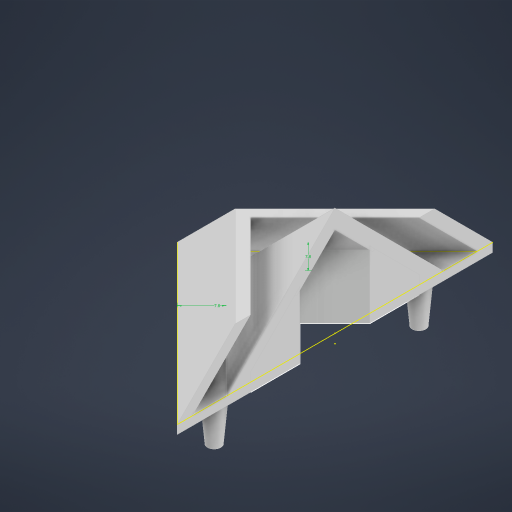
# Autodesk Inventor part: coltar5mmV3_notop
Saved by Autodesk Inventor 2023 (Build 270158000, 158)
## iProperties
Created: 2022-02-13
Part Number: coltar5mmV3_notop
Material: Generic
Document SubType Name: Modeling
Designer: Vlasciar
Density: 1 g/cm^3
Appearance: Default
Author: Vlasciar
Autodesk Inventor part; units mm, degrees
ref_plane "YZ Plane" through (0, 0, 0) normal (1, 0, 0) x (0, 1, 0)
ref_plane "XZ Plane" through (0, 0, 0) normal (0, 1, 0) x (-1, 0, 0)
ref_plane "XY Plane" through (0, 0, 0) normal (0, 0, 1) x (1, 0, 0)
sketch "Sketch2" plane through (0, 0, 0) normal (0, 1, 0) x (-1, 0, 0)
  line L0 (0, 35.355) -> (35.3557, 0)
  line L1 (35.3557, 0) -> (0, -35.355)
  line L2 (0, -35.355) -> (0, 35.355)
  point P0 (0, 0)
  point P1 (0, 0)
  dimension "d1" = 50
  dimension "d41" = 70.71
  constraints: 6 end point, 1 coincident, 1 equal length, 1 horizontal alignment, 1 midpoint
  measures "d1" distance of L0.start L0.end
  measures "d41" distance of L1.end L0.start
extrude "Extrusion1" add sketch "Sketch2" against normal blind 2
sketch "Sketch3" plane through (0, 0, 0) normal (0, 1, 0) x (1, 0, 0)
  line L0 (-35.3557, 0) -> (0, -35.355) projected
  line L1 (0, -35.355) -> (0, 35.355) projected
  line L2 (0, 35.355) -> (-35.3557, 0) projected
  point P0 (0, 0)
sketch "Sketch12" plane through (0, 0, 35.355) normal (1, 0, 0) x (0, 0, -1)
  line L0 (0, 0) -> (70.71, 0) projected
  line L1 (0, 0) -> (35.355, 35.3557)
  line L2 (35.355, 35.3557) -> (70.71, 0)
  line L3 (11.0308, 0) -> (59.6792, 0)
  line L4 (59.6792, 0) -> (35.355, 24.3247)
  line L5 (35.355, 24.3247) -> (11.0308, 0)
  point P0 (35.355, 0)
  point P1 (11.0308, 0)
  point P2 (59.6792, 0)
  dimension "d42" = 50
  dimension "d43" = 50
  dimension "d46" = 0
  dimension "d47" = 7.8
  dimension "d48" = 7.8
  constraints: 10 end point, 2 parallel, 1 horizontal
  measures "d42" distance of L1.end L0.end
  measures "d43" distance of L0.start L1.end
  measures "d46" distance between parallel lines of L0 L3
  measures "d47" distance between parallel lines of L2 L4
  measures "d48" distance between parallel lines of L1 L5
ref_plane "Work Plane5" through (-35.3557, 0, 0) normal (-0.5773466, 0.5773466, 0.5773577) x (0.7071136, 0, 0.7071)
ref_plane "Work Plane6" through (0, 0, -35.355) normal (0.5773466, -0.5773466, 0.5773577) x (-0.7071136, 0, 0.7071)
extrude "Extrusion10" add sketch "Sketch12" along normal up to surface surface through (-35.3557, 0, 0) normal (-0.5773466, 0.5773466, 0.5773577)
split "Split3" plane through (0, 0, -35.355) removes the side toward (-0.5773466, 0.5773466, -0.5773577)
shell "Shell3" thickness 2 removed faces 1 at (0, 11.7852, 0)
sketch "Sketch13" plane through (0, 0, 31.8909) normal (0, 1, 0) x (1, 0, 0)
  line L0 (-31.8916, 31.8909) -> (0, 0) projected
  line L1 (0, 63.7819) -> (0, 0) projected
  line L2 (0, 63.7819) -> (-31.8916, 31.8909) projected
  line L3 (0, 67.2459) -> (0, -3.4641) projected
  line L4 (0, 7.5667) -> (-24.3247, 31.8909)
  line L5 (-24.3247, 31.8909) -> (0, 56.2152)
  line L6 (0, -3.4641) -> (-35.3557, 31.8909) projected
  line L7 (-35.3557, 31.8909) -> (0, 67.2459) projected
  point P0 (0, 31.8909)
  dimension "d52" = 7.8
  dimension "d53" = 7.8
  constraints: 4 end point, 2 parallel, 2 point on line
  measures "d52" distance between parallel lines of L4 L6
  measures "d53" distance between parallel lines of L7 L5
ref_plane "Work Plane9" through (0, 24.3247, 0) normal (0.5773466, -0.5773466, -0.5773577) x (0, -0.7071136, 0.7071)
ref_plane "Work Plane10" through (0, 0, -24.3242) normal (-0.5773466, 0.5773466, -0.5773577) x (0, 0.7071136, 0.7071)
extrude "Extrusion18" add sketch "Sketch12" against normal up to surface separate body contours L5 L4 L0 surface through (0, 0, -24.3242) normal (-0.5773466, 0.5773466, -0.5773577)
split "Split5" plane through (0, 24.3247, 0) removes the side toward (-0.5773466, 0.5773466, 0.5773577) bodies 2
shell "Shell5" thickness 2 removed faces 1 at (0, 8.1082, 0) bodies 2
sketch "Sketch25" plane through (0, -2, 0) normal (0, -1, 0) x (1, 0, 0)
  line L0 (-18.8606, 0) -> (0, 18.8602) projected
  line L1 (0, -35.355) -> (0, 35.355) projected
  line L2 (0, 35.355) -> (-35.3557, 0) projected
  line L3 (-35.3557, 0) -> (0, -35.355) projected
  line L4 (0, -35.355) -> (0, 35.355) projected
  line L5 (0, -18.8602) -> (-18.8606, 0) projected
  point P0 (0, 0)
extrude "Extrusion24" cut sketch "Sketch25" against normal blind 2 contours L5 L1 L3 L2 L0 bodies 1
sketch "Sketch27" plane through (0, 0, 0) normal (0, -1, 0) x (1, 0, 0)
  line L0 (0, 35.355) -> (0, 31.8909) projected
  line L1 (-35.3557, 0) -> (0, 35.355) projected
  line L2 (0, -35.355) -> (-35.3557, 0) projected
  line L3 (0, -31.8909) -> (0, -35.355) projected
  line L4 (0, 35.355) -> (0, -35.355)
  line L5 (0, 0) -> (-35.3557, 0) projected
  line L6 (-35.3557, 0) -> (0, -35.355)
  line L7 (-35.3557, 0) -> (0, 35.355)
  line L8 (0, 18.8602) -> (-18.8606, 0) projected
  line L9 (0, 18.8602) -> (-18.8606, 0)
  line L10 (0, 24.3242) -> (0, -24.3242) projected
  line L11 (-18.8606, 0) -> (0, -18.8602)
  line L12 (0, -18.8602) -> (0, -35.355)
  point P0 (0, 31.8909)
  constraints: 12 end point, 3 collinear
extrude "Extrusion25" add sketch "Sketch27" along normal blind 2 contours L0 L4 L8 L5 L1 | L5 L11 L4 L3 L2 bodies 1
sketch "Sketch28" plane through (0, 2, 18.8602) normal (0, 1, 0) x (1, 0, 0)
  line L0 (0, 0) -> (-18.8606, 18.8602) projected
  line L1 (0, 37.7204) -> (0, 0) projected
  line L2 (-18.8606, 18.8602) -> (0, 37.7204) projected
  point P0 (0, 18.8602)
extrude "Extrusion26" cut sketch "Sketch28" against normal blind 10 bodies 2 1
sketch "Sketch29" plane through (0, -2, 0) normal (0, -1, 0) x (1, 0, 0)
  circle A0 centre (-4.0983, 22.9586) radius 1.5
  circle A1 centre (-4.0983, -22.9586) radius 1.5
  line L0 (0, 0) -> (-31.8916, 0) projected
  circle A2 centre (-26.4317, 0) radius 1.5
  dimension "d116" = 3
  dimension "d117" = 3
  dimension "d118" = 3
  constraints: 3 centre point, 1 point on line
  measures "d116" diameter of A0
  measures "d117" diameter of A1
  measures "d118" diameter of A2
extrude "Extrusion27" add sketch "Sketch29" along normal blind 10 bodies 1
draft "FaceDraft3" angle 5 pull direction (0, -1, 0) faces at (-2.6177, -8.6667, 22.718) (-2.6177, -8.6667, -23.1992) (-24.9511, -8.6667, -0.2406) fixed edges at (-5.5983, -12, 22.9586) (-5.5983, -12, -22.9586) (-27.9317, -12, 0)
ref_plane "Work Plane12" through (-9.1346, 13, 9.7258) normal (0, -1, 0) x (0.7071136, 0, 0.7071)
ref_plane "Work Plane11" through (-9.1346, -2, 9.7258) normal (0, -1, 0) x (0.7071136, 0, 0.7071)
sketch "Sketch30" plane through (-9.1346, 13, 9.7258) normal (0, -1, 0) x (0.7071136, 0, 0.7071)
  line L0 (27.2074, 21.2846) -> (-35.8048, 21.2846)
  line L1 (-35.8048, 21.2846) -> (-35.8048, -39.2765)
  line L2 (-35.8048, -39.2765) -> (27.2074, -39.2765)
  line L3 (27.2074, -39.2765) -> (27.2074, 21.2846)
  point P0 (-0.4179, -13.3363)
  constraints: 8 end point, 2 parallel, 1 horizontal, 1 perpendicular
extrude "Extrusion28" cut sketch "Sketch30" against normal blind 30 bodies 1 2
sketch "Sketch31" plane through (0, -2, 0) normal (0, -1, 0) x (1, 0, 0)
  line L0 (0, -18.8602) -> (-18.8606, 0) projected
  line L1 (-18.8606, 0) -> (0, 18.8602) projected
  line L2 (0, 18.8602) -> (0, 7.8604) projected
  line L3 (0, 18.8602) -> (0, 7.8604)
  line L4 (-7.8606, 0) -> (0, 7.8604) projected
  line L5 (0, 7.8604) -> (-7.8606, 0)
  line L6 (0, -7.8604) -> (-7.8606, 0) projected
  line L7 (-7.8606, 0) -> (0, -7.8604)
  line L8 (0, -7.8604) -> (0, -18.8602)
  line L9 (-18.8606, 0) -> (0, -18.8602)
  line L10 (-18.8606, 0) -> (0, 18.8602)
  line L11 (-18.8606, 0) -> (-7.8606, 0)
  point P0 (0, 0)
  constraints: 14 end point, 2 point on line, 1 collinear, 1 horizontal, 1 parallel
extrude "Extrusion29" add sketch "Sketch31" against normal up to surface contours L1 L2 L4 L11 surface through (-6.9534, 6.9534, 6.9536) normal (0.5773466, -0.5773466, -0.5773577) bodies 1
extrude "Extrusion30" add sketch "Sketch31" against normal up to surface contours L0 L11 L6 L8 surface through (-11.0077, 11.0077, 1.1547) normal (-0.5773466, 0.5773466, -0.5773577) bodies 1
sketch "Sketch33" plane through (-24.3247, 0, 0) normal (-0.5773466, 0.5773466, 0.5773577) x (0.7071136, 0, 0.7071)
  line L0 (25.2079, 15.9216) -> (9.1925, 15.9216) projected
  line L1 (9.1925, 15.9216) -> (14.1925, 24.5819)
  line L2 (25.2079, 15.9216) -> (20.208, 24.5819)
  line L3 (20.208, 24.5819) -> (14.1925, 24.5819)
  point P0 (17.2003, 9.9304)
  dimension "d129" = 10
  constraints: 6 end point, 1 horizontal
  measures "d129" distance of L0.end L1.end
sketch "Sketch34" plane through (0, 0, -24.3242) normal (-0.5773466, 0.5773466, -0.5773577) x (-0.7071136, 0, 0.7071)
  line L0 (25.2075, 15.9216) -> (9.1921, 15.9216) projected
  line L1 (9.1921, 15.9216) -> (11.6416, 17.3358) projected
  line L2 (9.1921, 15.9216) -> (14.192, 24.5819)
  line L3 (14.192, 24.5819) -> (20.2074, 24.5819)
  line L4 (20.2074, 24.5819) -> (25.2075, 15.9216)
  line L5 (25.2072, 25.1681) -> (25.2075, 15.9216) projected
  line L6 (25.2075, 15.9216) -> (9.1921, 15.9216)
  point P0 (17.1997, 9.9304)
  dimension "d130" = 10
  constraints: 8 end point, 1 collinear, 1 horizontal, 1 perpendicular
  measures "d130" distance of L0.end L2.end
extrude "Extrusion31" add sketch "Sketch33" against normal blind 2.45 bodies 2
extrude "Extrusion32" add sketch "Sketch34" against normal blind 2.45 bodies 2
sketch "Sketch35" plane through (0, 0, 35.355) normal (1, 0, 0) x (0, 0, -1)
  line L0 (19.9835, 25.4931) -> (55.8628, 25.4931)
  line L1 (55.8628, 25.4931) -> (55.8628, -4.2384)
  line L2 (55.8628, -4.2384) -> (19.9835, -4.2384)
  line L3 (19.9835, -4.2384) -> (19.9835, 25.4931)
  point P0 (35.355, 0)
  constraints: 8 end point, 2 parallel, 1 horizontal, 1 perpendicular
extrude "Extrusion33" cut sketch "Sketch35" along normal blind 2.45 bodies 2
sketch "Sketch37" plane through (0, 0, -24.3242) normal (-0.5773466, 0.5773466, -0.5773577) x (-0.7071136, 0, 0.7071)
  line L0 (20.2074, 24.5819) -> (14.192, 24.5819) projected
  line L1 (14.192, 24.5819) -> (17.8949, 30.9957)
  line L2 (20.2074, 24.5819) -> (16.715, 30.631)
  point P0 (17.1997, 9.9304)
  point P1 (17.1997, 29.7915)
  constraints: 4 end point
extrude "Extrusion34" add sketch "Sketch37" against normal blind 2.45 bodies 2
sketch "Sketch38" plane through (-24.3247, 0, 0) normal (-0.5773466, 0.5773466, 0.5773577) x (0.7071136, 0, 0.7071)
  line L0 (20.208, 24.5819) -> (14.1925, 24.5819) projected
  line L1 (20.208, 24.5819) -> (18.2076, 24.5819) projected
  line L2 (20.208, 24.5819) -> (17.2003, 29.7915)
  line L3 (14.1925, 24.5819) -> (17.2003, 29.7915) projected
  line L4 (14.1925, 24.5819) -> (17.2003, 29.7915)
  line L5 (20.208, 24.5819) -> (14.1925, 24.5819)
  point P0 (17.2003, 9.9304)
  constraints: 7 end point, 1 collinear
extrude "Extrusion35" add sketch "Sketch38" against normal blind 2.45 bodies 2
sketch "Sketch39" plane through (0, 0, 35.355) normal (1, 0, 0) x (0, 0, -1)
  line L0 (27.346, 17.253) -> (42.2787, 17.253)
  line L1 (42.2787, 17.253) -> (42.2787, 25.2793)
  line L2 (42.2787, 25.2793) -> (27.346, 25.2793)
  line L3 (27.346, 25.2793) -> (27.346, 17.253)
  point P0 (35.355, 0)
  constraints: 8 end point, 2 parallel, 1 horizontal, 1 perpendicular
extrude "Extrusion36" cut sketch "Sketch39" along normal blind 2.45 bodies 2
body "Solid1"
body "Solid4"
